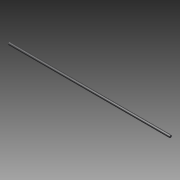
# Autodesk Inventor part: BNT 2010-2.61200 Shaft
Saved by Autodesk Inventor 2011 SP1 (Build 150282100, 282)
## iProperties
Created: 2017-05-16
Part Number: BNT 2010-2.61200 Shaft
Catalog Web Link: www.cadenas.de
Description: BNT Shaft-
Vendor: THK
Document SubType Name: Modeling
Designer: psAdmin
Manufacturer: THK
Mass: 398.248 g
Surface Area: 806.703 cm^2
Volume: 398.248 cm^3
Density: 1 g/cm^3
Category: PARTsolutions
Company: THK
Title: BNT 2010-2.61200 Shaft
Author: Cadenas PARTsolutions
PSOL_IDENT_0: {$CADENAS_DATA\23d-libs\thk\fed_screw\ball_screw\ball_screw\standard_lead_rbs\bnt\bnt_shaft.prj},198
PSOL_IDENT_1: {VTYP=3D},{NB=BNT 2010-2.61200 Shaft},{LINA=BNT 2010-2.61200 Shaft},{NN=BNT Shaft},{DATE=22.08.2011
PSOL_IDENT_2: 07:52:00},{GEOMDATE=22.08.2011 05:57:00},{VERSION=},{LINEID=520},{LINESUBID=-1},{WBVAR=ST,FS,SS}  {
PSOL_IDENT_3: NB=BNT 2010-2.61200 Shaft},{LINA=BNT 2010-2.61200 Shaft},{KT=DUMMY},{MN=BNT 2010-2.6},{ST=1200},{FS=
PSOL_IDENT_4: },{SS=},{OL=1268},{EL=2102},{L=58},{R1=11.300},{R2=11.300},{T1=2.500},{T2=2.500},{P3=16.000},{P4=16.
PSOL_IDENT_5: 000},{B3=14.300},{B4=14.300},{G2=4.000},{G3=1.150},{G4=1.150},{F3=10.150},{F4=10.150},{A3=15.000},{A
PSOL_IDENT_6: 4=15.000},{G1=4.000},{S1=12.000},{S2=13.000},{A1=15.000},{A2=15.000},{B1=12.000},{B2=12.000},{J1=16.
PSOL_IDENT_7: 000},{SD=20},{J2=16.000},{M1=15.000},{M2=15.000},{P11=1.000},{P2=1.000},{P1=2.500},{FSX='','None','-
PSOL_IDENT_8: H1','Type_H1','-H2','Type_H2','-H3','Type_H3','-J1','Type_J1','-J2','Type_J2','-J3','Type_J3'},{E3=1
PSOL_IDENT_9: 3},{E4=13},{F1=20},{E1=40},{N1=6},{H1=9},{F2=20},{E2=49},{N2=6},{H2=9},{STX=2044},{FSX1=0},{SSX1=0},
PSOL_IDENT_10: {VERMN=1},{VERK=1}
NN: BNT Shaft
NB: BNT 2010-2.61200 Shaft
NBSYN: $MN.$ST.$FS.$SS. Shaft
LINA: BNT 2010-2.61200 Shaft
MN: BNT 2010-2.6
ST: 1200
EL: 2102
L: 58
R1: 11.300
R2: 11.300
T1: 2.500
T2: 2.500
P3: 16.000
P4: 16.000
B3: 14.300
B4: 14.300
G2: 4.000
G3: 1.150
G4: 1.150
F3: 10.150
F4: 10.150
A3: 15.000
A4: 15.000
G1: 4.000
S1: 12.000
S2: 13.000
A1: 15.000
A2: 15.000
B1: 12.000
B2: 12.000
J1: 16.000
SD: 20
J2: 16.000
M1: 15.000
M2: 15.000
P11: 1.000
P2: 1.000
P1: 2.500
FSX: '','None','-H1','Type_H1','-H2','Type_H2','-H3','Type_H3','-J1','Type_J1','-J2','Type_J2','-J3','Type_J3'
E3: 13
E4: 13
F1: 20
E1: 40
N1: 6
H1: 9
F2: 20
E2: 49
N2: 6
H2: 9
VERMN: 1
SUPPLIER: THK
ARTICLENO: BNT 2010-2.61200 Shaft
BOMINFO: BNT 2010-2.61200 Shaft
CREATOR: CADENAS GmbH
Autodesk Inventor part; units mm, degrees
ref_plane "YZ Plane" through (0, 0, 0) normal (1, 0, 0) x (0, 1, 0)
ref_plane "XZ Plane" through (0, 0, 0) normal (0, 1, 0) x (-1, 0, 0)
ref_plane "XY Plane" through (0, 0, 0) normal (0, 0, 1) x (1, 0, 0)
sketch "Sketch_1" plane through (0, 0, 0) normal (0, 0, 1) x (1, 0, 0)
  line L0 (1263, 0) -> (5, 0)
  line L1 (5, 0) -> (5, 10)
  line L2 (5, 10) -> (1263, 10)
  line L3 (1263, 10) -> (1263, 0)
  line L4 (1263, 0) -> (5, 0)
  constraints: 10 end point
revolve "Revolution1" add sketch "Sketch_1" angle 360 about axis through (1263, 0, 0) along (1, 0, 0)
thread "Thread1" size "M20x2.5" class "6g" standard "ISO Metric profile" full length
sketch "Sketch_2" plane through (0, 0, 0) normal (0, 1, 0) x (-1, 0, 0)
  line L0 (-5, 0) -> (0, 0)
  line L1 (0, 0) -> (0, -9)
  line L2 (0, -9) -> (-1, -10)
  line L3 (-1, -10) -> (-4.8, -10)
  line L4 (-4.8, -10) -> (-4.8, -8)
  line L5 (-4.8, -8) -> (-5, -8)
  line L6 (-5, -8) -> (-5, 0)
  line L7 (-5, 0) -> (0, 0)
  constraints: 16 end point
revolve "Revolution2" add sketch "Sketch_2" angle 360 about axis through (5, 0, 0) along (1, 0, 0)
sketch "Sketch_3" plane through (0, 0, 0) normal (0, 1, 0) x (-1, 0, 0)
  line L0 (-1268, 0) -> (-1263, 0)
  line L1 (-1263, 0) -> (-1263, -8)
  line L2 (-1263, -8) -> (-1263.2, -8)
  line L3 (-1263.2, -8) -> (-1263.2, -10)
  line L4 (-1263.2, -10) -> (-1267, -10)
  line L5 (-1267, -10) -> (-1268, -9)
  line L6 (-1268, -9) -> (-1268, 0)
  line L7 (-1268, 0) -> (-1263, 0)
  constraints: 16 end point
revolve "Revolution3" add sketch "Sketch_3" angle 360 about axis through (1268, 0, 0) along (1, 0, 0)
ref_plane "bnt_s_1_XY" through (0, 0, 0) normal (-1, 0, 0) x (0, 0, -1)
ref_plane "bnt_s_1_YZ" through (0, 0, 0) normal (0, 0, -1) x (0, -1, 0)
ref_plane "bnt_s_1_ZX" through (0, 0, 0) normal (0, -1, 0) x (-1, 0, 0)
body "Solid1"
